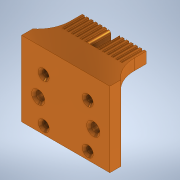
# Autodesk Inventor part: Soporte Motor X
Saved by Autodesk Inventor 2021 (Build 250183000, 183)
## iProperties
Created: 2023-01-28
Part Number: Soporte Motor X
Material: Oro
Document SubType Name: Modeling
Designer: Diego.labarca
Density: 19.3 g/cm^3
Appearance: Metal 1600F
Author: Diego.labarca
Autodesk Inventor part; units mm, degrees
ref_plane "YZ Plane" through (0, 0, 0) normal (1, 0, 0) x (0, 1, 0)
ref_plane "XZ Plane" through (0, 0, 0) normal (0, 1, 0) x (-1, 0, 0)
ref_plane "XY Plane" through (0, 0, 0) normal (0, 0, 1) x (1, 0, 0)
sketch "Boceto1" plane through (0, 0, 0) normal (0, 0, 1) x (1, 0, 0)
  line L0 (-20, 12.5) -> (20, 12.5)
  line L1 (20, 12.5) -> (20, -12.5)
  line L2 (20, -12.5) -> (-20, -12.5)
  line L3 (-20, -12.5) -> (-20, 12.5)
  line L4 (4.8304, 0) -> (0, 0)
  line L5 (0, 0) -> (0, 3.5516)
  dimension "d2" = 40
  dimension "d3" = 25
  constraints: 12 end point, 2 horizontal, 2 parallel, 2 perpendicular, 2 other
  measures "d2" distance of L1.end L2.end
  measures "d3" distance of L0.end L1.end
extrude "Extrusión1" add sketch "Boceto1" along normal blind 5
sketch "Boceto2" plane through (0, 0, 5) normal (0, 0, 1) x (1, 0, 0)
  circle A0 centre (10, 10) radius 1.5
  point P0 (0, 0)
  dimension "d6" = 3
  dimension "d7" = 10
  dimension "d8" = 10
  constraints: 1 centre point
  measures "d6" diameter of A0
  measures "d7" horizontal distance of point (0, 0) A0.centre
  measures "d8" horizontal distance of point (0, 0) A0.centre
extrude "Extrusión2" cut sketch "Boceto2" against normal through all
pattern_linear "Patrón rectangular1" count 2 spacing 20 along (0, -1, 0) count 2 spacing 20 along (-1, 0, 0) of "Extrusión2"
sketch "Boceto3" plane through (0, 0, 5) normal (0, 0, 1) x (1, 0, 0)
  circle A0 centre (12.5, 0) radius 2
  circle A1 centre (-12.5, 0) radius 2
  line L0 (-20, 12.5) -> (-20, -12.5) projected
  point P0 (0, 0)
  dimension "d17" = 4
  dimension "d18" = 0
  dimension "d19" = 12.5
  dimension "d20" = 4
  dimension "d21" = 0
  dimension "d23" = 12.5
  constraints: 2 centre point
  measures "d17" diameter of A0
  measures "d18" vertical distance of point (0, 0) A0.centre
  measures "d19" distance of point (0, 0) A0.centre
  measures "d20" diameter of A1
  measures "d21" vertical distance of point (0, 0) A1.centre
  measures "d23" distance of point (0, 0) A1.centre
extrude "Extrusión3" cut sketch "Boceto3" against normal through all
sketch "Boceto4" plane through (20, -12.5, 0) normal (1, 0, 0) x (0, 0, -1)
  line L0 (0, 25) -> (-5, 25) projected
  line L1 (-5, 25) -> (0, 25)
  line L2 (0, 25) -> (0, 33)
  line L3 (0, 33) -> (-5, 33)
  line L4 (-5, 33) -> (-5, 25)
  line L5 (0, 33) -> (17, 33)
  line L6 (17, 33) -> (17, 28)
  line L7 (17, 28) -> (0, 28)
  line L8 (0, 28) -> (0, 33)
  line L9 (0, 0) -> (0, 25) projected
  line L10 (-5, 0) -> (-5, 25) projected
  point P0 (0, 12.5)
  point P1 (0, 28)
  dimension "d26" = 17
  dimension "d27" = 5
  dimension "d28" = 8
  constraints: 16 end point, 4 parallel, 2 collinear, 2 horizontal, 2 perpendicular
  measures "d26" distance of L6.end L7.end
  measures "d27" distance of L5.end L6.end
  measures "d28" distance of L3.end L0.end
extrude "Extrusión4" add sketch "Boceto4" against normal up to surface (40 mm away)
sketch "Boceto5" plane through (20, 15.5, -17) normal (0, -1, 0) x (1, 0, 0)
  line L0 (0, 0) -> (-40, 0) projected
  line L1 (-20, 0) -> (-18.5, 0)
  line L2 (-18.5, 0) -> (-18.5, 10)
  line L3 (-18.5, 10) -> (-20, 10)
  line L4 (-20, 10) -> (-20, 0)
  point P0 (-20, 17)
  point P1 (-18.5, 0)
  dimension "d31" = 1.5
  dimension "d32" = 10
  constraints: 8 end point, 2 parallel, 1 horizontal, 1 midpoint, 1 perpendicular
  measures "d31" distance of L3.end L2.end
  measures "d32" distance of L2.end L1.end
extrude "Extrusión5" cut sketch "Boceto5" against normal up to surface (5 mm away)
sketch "Boceto6" plane through (20, 15.5, -17) normal (0, 0, -1) x (1, 0, 0)
  line L0 (0, 0) -> (-40, 0) projected
  line L1 (-17.4489, 0) -> (-16.4489, 0)
  line L2 (-16.4489, 0) -> (-16.4489, -0.6)
  line L3 (-16.4489, -0.6) -> (-17.4489, -0.6)
  line L4 (-17.4489, -0.6) -> (-17.4489, 0)
  line L5 (0, -5) -> (-18.5, -5) projected
  line L6 (-17.4489, -5) -> (-16.4489, -5)
  line L7 (-16.4489, -5) -> (-16.4489, -4.4)
  line L8 (-16.4489, -4.4) -> (-17.4489, -4.4)
  line L9 (-17.4489, -4.4) -> (-17.4489, -5)
  line L10 (-15.4489, 0) -> (-14.4489, 0)
  line L11 (-14.4489, 0) -> (-14.4489, -0.6)
  line L12 (-14.4489, -0.6) -> (-15.4489, -0.6)
  line L13 (-15.4489, -0.6) -> (-15.4489, 0)
  line L14 (-15.4489, -5) -> (-14.4489, -5)
  line L15 (-14.4489, -5) -> (-14.4489, -4.4)
  line L16 (-14.4489, -4.4) -> (-15.4489, -4.4)
  line L17 (-15.4489, -4.4) -> (-15.4489, -5)
  line L18 (-13.4489, 0) -> (-12.4489, 0)
  line L19 (-12.4489, 0) -> (-12.4489, -0.6)
  line L20 (-12.4489, -0.6) -> (-13.4489, -0.6)
  line L21 (-13.4489, -0.6) -> (-13.4489, 0)
  line L22 (-13.4489, -5) -> (-12.4489, -5)
  line L23 (-12.4489, -5) -> (-12.4489, -4.4)
  line L24 (-12.4489, -4.4) -> (-13.4489, -4.4)
  line L25 (-13.4489, -4.4) -> (-13.4489, -5)
  line L26 (-11.4489, 0) -> (-10.4489, 0)
  line L27 (-10.4489, 0) -> (-10.4489, -0.6)
  line L28 (-10.4489, -0.6) -> (-11.4489, -0.6)
  line L29 (-11.4489, -0.6) -> (-11.4489, 0)
  line L30 (-11.4489, -5) -> (-10.4489, -5)
  line L31 (-10.4489, -5) -> (-10.4489, -4.4)
  line L32 (-10.4489, -4.4) -> (-11.4489, -4.4)
  line L33 (-11.4489, -4.4) -> (-11.4489, -5)
  line L34 (-9.4489, 0) -> (-8.4489, 0)
  line L35 (-8.4489, 0) -> (-8.4489, -0.6)
  line L36 (-8.4489, -0.6) -> (-9.4489, -0.6)
  line L37 (-9.4489, -0.6) -> (-9.4489, 0)
  line L38 (-9.4489, -5) -> (-8.4489, -5)
  line L39 (-8.4489, -5) -> (-8.4489, -4.4)
  line L40 (-8.4489, -4.4) -> (-9.4489, -4.4)
  line L41 (-9.4489, -4.4) -> (-9.4489, -5)
  line L42 (-7.4489, 0) -> (-6.4489, 0)
  line L43 (-6.4489, 0) -> (-6.4489, -0.6)
  line L44 (-6.4489, -0.6) -> (-7.4489, -0.6)
  line L45 (-7.4489, -0.6) -> (-7.4489, 0)
  line L46 (-7.4489, -5) -> (-6.4489, -5)
  line L47 (-6.4489, -5) -> (-6.4489, -4.4)
  line L48 (-6.4489, -4.4) -> (-7.4489, -4.4)
  line L49 (-7.4489, -4.4) -> (-7.4489, -5)
  point P0 (-16.4489, -5)
  point P1 (-16.4489, 0)
  point P2 (-14.4489, 0)
  point P3 (-15.4489, 0)
  point P4 (-15.4489, -5)
  point P5 (-14.4489, -5)
  point P6 (-13.4489, -5)
  point P7 (-12.4489, -5)
  point P8 (-12.4489, 0)
  point P9 (-13.4489, 0)
  point P10 (-10.4489, 0)
  point P11 (-11.4489, 0)
  point P12 (-11.4489, -5)
  point P13 (-10.4489, -5)
  point P14 (-9.4489, -5)
  point P15 (-8.4489, -5)
  point P16 (-8.4489, 0)
  point P17 (-9.4489, 0)
  point P18 (-7.4489, -5)
  point P19 (-6.4489, -5)
  point P20 (-6.4489, 0)
  point P21 (-7.4489, 0)
  dimension "d64" = 1
  dimension "d65" = 0.6
  dimension "d66" = 0.6
  dimension "d69" = 2
  constraints: 96 end point, 14 point on line, 4 parallel, 3 horizontal, 2 perpendicular, 80 other
  measures "d64" distance of L2.end L3.end
  measures "d65" distance of L1.end L2.end
  measures "d66" distance of L7.end L6.end
  measures "d69" distance of L1.start L10.start
extrude "Extrusión6" cut sketch "Boceto6" against normal up to surface (10 mm away)
fillet "Empalme1" radius 1.5 2 edges at (1.5, 15.5, -12) (1.5, 20.5, -12)
sketch "Boceto8" plane through (20, 15.5, -17) normal (0, -1, 0) x (1, 0, 0)
  line L0 (0, 17) -> (0, 0) projected
  line L1 (0, 0) -> (-5.5, 0)
  line L2 (-5.5, 0) -> (-5.5, 17)
  line L3 (-5.5, 17) -> (0, 17)
  line L4 (0, 17) -> (0, 0)
  line L5 (-40, 17) -> (0, 17) projected
  point P0 (-20, 17)
  point P1 (0, 17)
  dimension "d52" = 5.5
  constraints: 8 end point, 2 parallel, 1 collinear, 1 horizontal, 1 perpendicular
  measures "d52" distance of L2.end L3.end
extrude "Extrusión8" cut sketch "Boceto8" against normal through all
fillet "Empalme2" radius 15 1 edges at (14.5, 18, 0)
mirror "Simetría2" about plane through (0, 0, 0) normal (1, 0, 0) of "Extrusión5", "Extrusión6", "Empalme1", "Extrusión8", "Empalme2"
fillet "Empalme4" radius 2 1 edges at (0, 15.5, 0)
sketch "Boceto11" plane through (0, 0, 0) normal (0, 0, -1) x (-1, 0, 0)
  line L0 (20, -12.5) -> (-20, -12.5) projected
  line L1 (-20, -12.5) -> (20, -12.5)
  line L2 (20, -12.5) -> (20, -13.5)
  line L3 (20, -13.5) -> (-20, -13.5)
  line L4 (-20, -13.5) -> (-20, -12.5)
  point P0 (0, 0)
  dimension "d74" = 1
  constraints: 8 end point, 2 parallel, 1 horizontal, 1 perpendicular
  measures "d74" distance of L1.end L2.end
extrude "Extrusión11" add sketch "Boceto11" against normal up to surface (5 mm away)
chamfer "Chaflán1" distance 1 angle 45 6 edges at (-11.5, 10, 5) (8.5, 10, 5) (10.5, 0, 5) (-14.5, 0, 5) (-11.5, -10, 5) (8.5, -10, 5)
equation "\"d20\" = d17"
equation "\"d23\" = d19"
